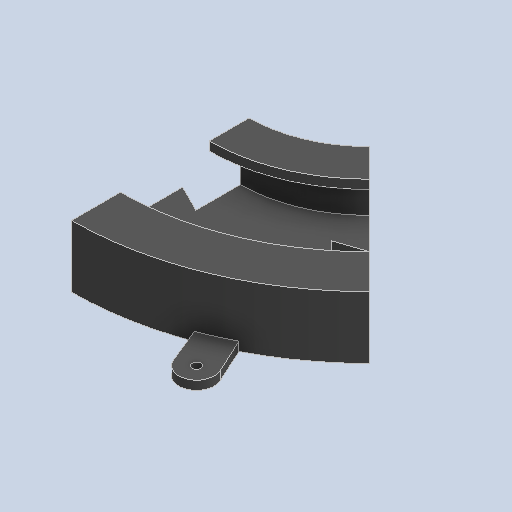
# Autodesk Inventor part: Carousel Fixed Track
Saved by Autodesk Inventor 2023 (Build 270158000, 158)
## iProperties
Created: 2022-11-03
Part Number: Carousel Fixed Track
Material: PLA Plastic
Document SubType Name: Modeling
Designer: cheng
Density: 1.25002 g/cm^3
Appearance: Generic
Mass: 955.709 g
Surface Area: 1679.01 cm^2
Volume: 764.553 cm^3
Author: cheng
Autodesk Inventor part; units mm, degrees
ref_plane "YZ Plane" through (0, 0, 0) normal (1, 0, 0) x (0, 1, 0)
ref_plane "XZ Plane" through (0, 0, 0) normal (0, 1, 0) x (-1, 0, 0)
ref_plane "XY Plane" through (0, 0, 0) normal (0, 0, 1) x (1, 0, 0)
sketch "Sketch1" plane through (0, 0, 0) normal (0, 1, 0) x (-1, 0, 0)
  circle A0 centre (0, 0) radius 335
  line L0 (335, 0) -> (-335, 0)
  line L1 (0, -335) -> (0, 335)
  line L2 (0, 0) -> (-236.8808, 236.8808)
  line L3 (0, 0) -> (236.8808, -236.8808)
  line L4 (0, 0) -> (236.8808, 236.8808)
  line L5 (0, 0) -> (-236.8808, -236.8808)
  circle A1 centre (0, 0) radius 135
  point P0 (-95.4594, 95.4594)
  point P1 (0, 135)
  dimension "d0" = 670
  dimension "d1" = 45
  dimension "d2" = 45
  dimension "d17" = 200
  constraints: 12 end point, 2 coincident, 2 collinear, 1 centre point, 1 horizontal, 10 other
  measures "d1" angle of L1 L3
  measures "d2" angle of L5 L1
extrude "Extrusion1" add sketch "Sketch1" along normal blind 70 contours L1 A1 L2 A0
sketch "Sketch2" plane through (95.4594, 0, 95.4594) normal (0.7071068, 0, -0.7071068) x (-0.7071068, 0, -0.7071068)
  line L0 (-190, 60) -> (-10, 60)
  line L1 (-10, 60) -> (-10, 10)
  line L2 (-10, 10) -> (-190, 10)
  line L3 (-190, 10) -> (-190, 60)
  line L4 (-200, 0) -> (0, 0) projected
  line L5 (-200, 70) -> (0, 70) projected
  line L6 (-200, 0) -> (-200, 70) projected
  line L7 (0, 0) -> (0, 70) projected
  point P0 (135, 0)
  point P1 (0, 35)
  dimension "d6" = 10
  dimension "d7" = 10
  dimension "d8" = 10
  dimension "d9" = 10
  constraints: 8 end point, 2 parallel, 1 horizontal, 1 midpoint, 1 perpendicular
  measures "d6" distance between parallel lines of L4 L2
  measures "d7" distance between parallel lines of L5 L0
  measures "d8" distance between parallel lines of L6 L3
  measures "d9" distance from line of point (0, 35) L1
sketch3d "3D Sketch1"
  arc A0 (95.4594, 70, 95.4594) -> (0, 70, 135) centre (0, 70, 0) ccw
sweep "Sweep1" cut profiles "Sketch2" path "3D Sketch1" contours L0 L1 L2 L3
sketch "Sketch3" plane through (95.4594, 0, 95.4594) normal (0.7071068, 0, -0.7071068) x (-0.7071068, 0, -0.7071068)
  line L0 (-101.8808, 70) -> (-200, 70) projected
  line L1 (32.4695, 60) -> (-94.8097, 60) projected
  line L2 (-145, 70) -> (-45, 70)
  line L3 (-45, 70) -> (-45, 60)
  line L4 (-45, 60) -> (-145, 60)
  line L5 (-145, 60) -> (-145, 70)
  line L6 (-200, 0) -> (-200, 70) projected
  line L7 (0, 0) -> (0, 70) projected
  point P0 (135, 0)
  dimension "d16" = 100
  dimension "d18" = 45
  constraints: 8 end point, 2 parallel, 2 point on line, 1 horizontal, 1 perpendicular
  measures "d16" distance of L2.start L2.end
  measures "d18" distance between parallel lines of L7 L3
sketch3d "3D Sketch2"
  arc A0 (95.4594, 70, 95.4594) -> (0, 70, 135) centre (0, 70, 0) ccw
sweep "Sweep2" cut profiles "Sketch3" path "3D Sketch2"
sketch "Sketch5" plane through (0, 10, 325) normal (0, 1, 0) x (1, 0, 0)
  line L0 (0, 0) -> (0, 180) projected
  arc A0 (0, 145) -> (127.2792, 197.7208) centre (0, 325) ccw projected
  line L1 (127.2792, 197.7208) -> (95.4594, 229.5406) projected
  arc A1 (0, 190) -> (95.4594, 229.5406) centre (0, 325) ccw projected
  line L2 (0, 190) -> (0, 145) projected
  arc A2 (0, 45) -> (197.9899, 127.0101) centre (0, 325) ccw projected
  line L3 (0, 45) -> (0, -10) projected
  arc A3 (0, -10) -> (236.8808, 88.1192) centre (0, 325) ccw projected
  line L4 (236.8808, 88.1192) -> (197.9899, 127.0101) projected
  line L5 (0, 145) -> (-30, 145)
  line L6 (-30, 145) -> (-30, 44.996)
  line L7 (-30, 44.996) -> (0, 44.996)
  line L8 (0, 44.996) -> (0, 145)
  line L9 (0, 190) -> (0, -10) projected
  line L10 (0, 129.998) -> (-30, 129.998)
  line L11 (-30, 129.998) -> (-30, 59.998)
  line L12 (-30, 59.998) -> (0, 59.998)
  line L13 (0, 59.998) -> (0, 129.998)
  line L14 (0, 44.996) -> (-30, 145) construction
  line L15 (0, 145) -> (-30, 44.996) construction
  line L16 (0, 59.998) -> (-30, 129.998) construction
  line L17 (-30, 59.998) -> (0, 129.998) construction
  line L18 (-15, 94.998) -> (-30, 94.998) construction
  line L19 (-15, 94.998) -> (-30, 94.998) construction
  line L20 (0, 59.998) -> (-30, 44.996)
  line L21 (0, 129.998) -> (-30, 145)
  point P0 (0, 44.996)
  point P1 (0, 59.998)
  dimension "d21" = 30
  dimension "d27" = 70
  constraints: 32 end point, 5 equal length, 4 midpoint, 2 horizontal, 2 perpendicular, 2 point on line, 1 collinear
  measures "d21" distance between parallel lines of L11 L0
  measures "d27" distance between parallel lines of L10 L12
extrude "Extrusion2" add sketch "Sketch5" against normal blind 10 contours L6 L12 L20 | L12 L6 L10 L0 | L10 L6 L21
sketch "Sketch6" plane through (-30, 10, 280.004) normal (0, 1, 0) x (1, 0, 0)
  line L0 (132.5305, 177.4736) -> (259.8097, 50.1943) projected
  arc A0 (30, 135.004) -> (132.5305, 177.4736) centre (30, 280.004) ccw projected
  line L1 (30, 85.002) -> (30, 135.004) projected
  line L2 (0, 100.004) -> (0, 0) projected
  line L3 (30, -44.996) -> (30, 15.002) projected
  arc A1 (30, -44.996) -> (259.8097, 50.1943) centre (30, 280.004) ccw projected
  arc A2 (30, 100.004) -> (157.2792, 152.7248) centre (30, 280.004) ccw projected
  line L4 (157.2792, 152.7248) -> (136.066, 131.5116)
  line L5 (136.066, 131.5116) -> (206.7767, 60.8009)
  line L6 (206.7767, 60.8009) -> (227.9899, 82.0141)
  line L7 (227.9899, 82.0141) -> (157.2792, 152.7248)
  arc A3 (30, 100.004) -> (157.2792, 152.7248) centre (30, 280.004) ccw projected
  arc A4 (30, 0.004) -> (227.9899, 82.0141) centre (30, 280.004) ccw projected
  line L8 (30, 0.004) -> (30, -54.996) projected
  arc A5 (30, -54.996) -> (266.8808, 43.1233) centre (30, 280.004) ccw projected
  line L9 (266.8808, 43.1233) -> (227.9899, 82.0141) projected
  arc A6 (30, 100.004) -> (157.2792, 152.7248) centre (30, 280.004) ccw projected
  line L10 (157.2792, 152.7248) -> (125.4594, 184.5446) projected
  arc A7 (30, 145.004) -> (125.4594, 184.5446) centre (30, 280.004) ccw projected
  line L11 (30, 145.004) -> (30, 100.004) projected
  line L12 (167.8858, 142.1182) -> (146.6726, 120.905)
  line L13 (146.6726, 120.905) -> (196.1701, 71.4075)
  line L14 (196.1701, 71.4075) -> (217.3833, 92.6207)
  line L15 (217.3833, 92.6207) -> (167.8858, 142.1182)
  line L16 (167.8858, 142.1182) -> (196.1701, 71.4075) construction
  line L17 (217.3833, 92.6207) -> (146.6726, 120.905) construction
  line L18 (157.2792, 152.7248) -> (206.7767, 60.8009) construction
  line L19 (227.9899, 82.0141) -> (136.066, 131.5116) construction
  line L20 (182.028, 106.7629) -> (171.4214, 96.1563) construction
  line L21 (182.028, 106.7629) -> (171.4214, 96.1563) construction
  line L22 (217.3833, 92.6207) -> (206.7767, 60.8009)
  line L23 (167.8858, 142.1182) -> (136.066, 131.5116)
  line L24 (30, 85.002) -> (0, 100.004) projected
  line L25 (0, 0) -> (30, 15.002) projected
  point P0 (207.7219, 63.6364)
  point P1 (217.3833, 92.6207)
  point P2 (167.8858, 142.1182)
  point P3 (205.637, 61.9406)
  dimension "d23" = 30
  dimension "d24" = 70
  constraints: 32 end point, 6 collinear, 4 midpoint, 4 parallel, 3 perpendicular, 2 tangent
  measures "d23" distance between parallel lines of L13 L15
  measures "d24" distance between parallel lines of L12 L14
extrude "Extrusion3" cut sketch "Sketch6" against normal blind 10 contours L0 L14 L5 L12 | L12 L5 L23 | L22 A4 L5 L14 | L22 L5 A4
sketch "Sketch7" plane through (-30, 10, 280.004) normal (0, 1, 0) x (1, 0, 0)
  arc A0 (30, -44.996) -> (259.8097, 50.1943) centre (30, 280.004) ccw projected
  arc A1 (30, 0.004) -> (227.9899, 82.0141) centre (30, 280.004) ccw projected
  line L0 (30, 0.004) -> (30, -54.996) projected
  arc A2 (30, -54.996) -> (266.8808, 43.1233) centre (30, 280.004) ccw projected
  line L1 (266.8808, 43.1233) -> (227.9899, 82.0141) projected
  arc A3 (30, -54.996) -> (266.8808, 43.1233) centre (30, 280.004) ccw construction
  line L2 (30, 0.004) -> (266.8808, 43.1233) construction
  line L3 (266.8808, 43.1233) -> (227.9899, 82.0141) construction
  line L4 (266.8808, 43.1233) -> (217.3833, 92.6207) construction
  line L5 (227.9899, 82.0141) -> (227.9899, 82.0141) construction
  line L6 (217.3833, 92.6207) -> (259.8097, 50.1943) construction
  line L7 (227.9899, 82.0141) -> (227.9899, 82.0141) construction
  line L8 (227.9899, 82.0141) -> (227.9899, 82.0141) construction
  line L9 (227.9899, 82.0141) -> (227.9899, 82.0141) construction
  line L10 (227.9899, 82.0141) -> (39.9698, -54.8476) construction
  line L11 (143.7771, 20.7148) -> (196.6229, -99.7168) construction
  circle A4 centre (181.9243, -66.2198) radius 20
  line L12 (163.3808, -73.7121) -> (147.2566, -33.8047)
  line L13 (200.0777, -57.8259) -> (181.9244, -18.5659)
  circle A5 centre (181.9243, -66.2198) radius 5
  point P0 (181.9244, -18.5659)
  point P1 (147.2566, -33.8047)
  dimension "d28" = 40
  dimension "d31" = 10
  constraints: 20 end point, 6 point on circle, 4 point on line, 2 centre point, 2 tangent, 1 coincident, 1 collinear, 1 line through centre
  measures "d28" diameter of A4
  measures "d31" diameter of A5
extrude "Extrusion4" add sketch "Sketch7" against normal blind 10 contours A2 L13 A4 L12 | A4
body "Solid1"
